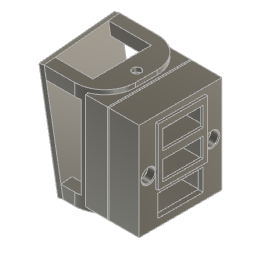
Lock Shoot v26 (Autodesk Fusion 360 design; units mm, degrees)
Autodesk Fusion 360 part; units mm, degrees
note: some values were not read from the file. Chosen so that the rebuilt part matches the saved one: which bodies a step acts on; which sketch regions a step uses; which face or edge a step refers to.
sketch "Sketch1" plane through (0, 0, 0) normal (1, 0, 0) x (0, 1, 0)
  line L0 (16, -20) -> (-16, -20)
  line L1 (-16, -20) -> (-16, 20)
  line L2 (-16, 20) -> (16, 20)
  line L3 (16, 20) -> (16, -20)
  line L4 (16, -20) -> (-16, 20) construction
  line L5 (-16, -20) -> (16, 20) construction
  line L6 (13, -0.5) -> (-13, -0.5)
  line L7 (-13, -0.5) -> (-13, 0.5)
  line L8 (-13, 0.5) -> (13, 0.5)
  line L9 (13, 0.5) -> (13, -0.5)
  line L10 (13, -0.5) -> (-13, 0.5) construction
  line L11 (-13, -0.5) -> (13, 0.5) construction
  circle A0 centre (13, 0) radius 1.6
  circle A1 centre (-13, 0) radius 1.6
  circle A2 centre (13, 0) radius 2.5
  circle A3 centre (-13, 0) radius 2.5
  line L12 (9.8559, -5.7872) -> (-9.8471, -5.7872)
  line L13 (-9.8471, -5.7872) -> (-9.8471, 17.1997)
  line L14 (-9.8471, 17.1997) -> (9.8559, 17.1997)
  line L15 (9.8559, 17.1997) -> (9.8559, -5.7872)
  line L16 (9.8559, -5.7872) -> (-9.8471, 17.1997) construction
  line L17 (-9.8471, -5.7872) -> (9.8559, 17.1997) construction
  line L18 (8.3025, -3.9749) -> (-8.3025, -3.9749)
  line L19 (-8.3025, -3.9749) -> (-8.3025, 3.9749)
  line L20 (-8.3025, 3.9749) -> (8.3025, 3.9749)
  line L21 (8.3025, 3.9749) -> (8.3025, -3.9749)
  line L22 (8.3025, -3.9749) -> (-8.3025, 3.9749) construction
  line L23 (-8.3025, -3.9749) -> (8.3025, 3.9749) construction
  line L24 (-8.3025, 7.0251) -> (-8.3025, 14.9749)
  line L25 (-8.3025, 14.9749) -> (8.3025, 14.9749)
  line L26 (8.3025, 14.9749) -> (8.3025, 7.0251)
  line L27 (8.3025, 7.0251) -> (-8.3025, 7.0251)
  line L28 (-9.3025, -8.0251) -> (9.3025, -8.0251)
  line L29 (-9.3025, -16.9749) -> (-9.3025, -8.0251)
  line L30 (9.3025, -16.9749) -> (-9.3025, -16.9749)
  line L31 (9.3025, -8.0251) -> (9.3025, -16.9749)
  line L32 (-8.3025, 14.9749) -> (-3.8025, 14.9749)
  line L33 (-3.8025, 14.9749) -> (-3.8025, 11)
  line L34 (-3.8025, 11) -> (-8.3025, 11)
  line L35 (-8.3025, 11) -> (-8.3025, 14.9749)
  line L36 (8.3025, 14.9749) -> (3.8025, 14.9749)
  line L37 (3.8025, 14.9749) -> (3.8025, 11)
  line L38 (3.8025, 11) -> (8.3025, 11)
  line L39 (8.3025, 11) -> (8.3025, 14.9749)
  circle A4 centre (-3.8025, 11) radius 2.5
  circle A5 centre (3.8025, 11) radius 2.5
  circle A6 centre (-3.8025, 0) radius 2.5
  circle A7 centre (3.8025, 0) radius 2.5
  line L40 (-9.3025, -8.0251) -> (-4.2025, -8.0251)
  line L41 (-4.2025, -8.0251) -> (-4.2025, -12.5)
  line L42 (-4.2025, -12.5) -> (-9.3025, -12.5)
  line L43 (-9.3025, -12.5) -> (-9.3025, -8.0251)
  line L44 (9.3025, -8.0251) -> (4.2025, -8.0251)
  line L45 (4.2025, -8.0251) -> (4.2025, -12.5)
  line L46 (4.2025, -12.5) -> (9.3025, -12.5)
  line L47 (9.3025, -12.5) -> (9.3025, -8.0251)
  circle A8 centre (-4.2025, -12.5) radius 2.5
  circle A9 centre (4.2025, -12.5) radius 2.55
  circle A10 centre (-13, 0) radius 2.85
  circle A11 centre (13, 0) radius 2.85
  point P0 (0.0044, 5.7062)
  dimension "d1" = 32
  dimension "d2" = 40
  dimension "d3" = 26
  dimension "d4" = 1
  dimension "d5" = 3.2
  dimension "d6" = 3.2
  dimension "d7" = 5
  dimension "d8" = 5
  dimension "d9" = 4.5
  dimension "d10" = 4.5
  dimension "d11" = 5
  dimension "d12" = 5
  dimension "d13" = 5
  dimension "d14" = 5
  dimension "d15" = 5.1
  dimension "d16" = 5.1
  dimension "d17" = 5
  dimension "d18" = 5.1
  dimension "d82" = 5.7
  dimension "d83" = 5.7
  constraint horizontal L0
  constraint perpendicular L0 L1
  constraint parallel L0 L2
  constraint parallel L1 L3
  constraint coincident L4 origin
  constraint coincident L5 origin
  constraint horizontal L6
  constraint perpendicular L6 L7
  constraint parallel L6 L8
  constraint parallel L7 L9
  constraint coincident L10 origin
  constraint coincident L11 origin
  constraint midpoint L9 A0.centre
  constraint midpoint L7 A1.centre
  constraint concentric A0 A2
  constraint concentric A1 A3
  constraint horizontal L12
  constraint perpendicular L12 L13
  constraint parallel L12 L14
  constraint parallel L13 L15
  constraint coincident L16 P0
  constraint coincident L17 P0
  constraint horizontal L18
  constraint perpendicular L18 L19
  constraint parallel L18 L20
  constraint parallel L19 L21
  constraint coincident L16 L18.start
  constraint coincident L22 origin
  constraint coincident L23 origin
  constraint horizontal L27
  constraint perpendicular L24 L27
  constraint parallel L25 L27
  constraint parallel L24 L26
  constraint horizontal L30
  constraint perpendicular L29 L30
  constraint parallel L28 L30
  constraint parallel L29 L31
  constraint horizontal L32
  constraint vertical L33
  constraint horizontal L34
  constraint vertical L35
  constraint horizontal L36
  constraint vertical L37
  constraint horizontal L38
  constraint vertical L39
  constraint coincident L33.end L34.start
  constraint coincident L37.end L38.start
  constraint horizontal L40
  constraint vertical L41
  constraint horizontal L42
  constraint vertical L43
  constraint horizontal L44
  constraint vertical L45
  constraint horizontal L46
  constraint vertical L47
  constraint coincident L41.end L42.start
  constraint coincident L45.end L46.start
  constraint concentric A1 A10
  constraint concentric A0 A11
  measures "d1" distance of L1.end L2.end
  measures "d2" distance of L0.end L1.end
  measures "d3" distance of L7.end L8.end
  measures "d4" distance of L6.end L7.end
  measures "d5" diameter of A0
  measures "d6" diameter of A1
  measures "d7" diameter of A2
  measures "d8" diameter of A3
  measures "d9" distance of L24.end L32.end
  measures "d10" distance of L25.end L36.end
  measures "d11" diameter of A4
  measures "d12" diameter of A5
  measures "d13" diameter of A6
  measures "d14" diameter of A7
  measures "d15" distance of L28.start L40.end
  measures "d16" distance of L28.end L44.end
  measures "d17" diameter of A8
  measures "d18" diameter of A9
  measures "d82" diameter of A10
  measures "d83" diameter of A11
extrude "Extrude1" add sketch "Sketch1" against normal blind 8 contours L0 L1 L2 L3 | L6 L8 A0 A2 | L6 L8 A0 A2 | L6 L8 A2 A11 | L6 L8 A2 A11 | L6 L8 L15 A11 | L6 L8 L13 A10 | L6 L8 A3 A10 | L6 L8 A3 A10 | L6 L8 A1 A3 | L6 L8 A1 A3 makes body 1
extrude "Extrude2" add sketch "Sketch1" along normal blind 1 separate body contours L6 L12 L13 L15 L18 L19 L21 | L6 L8 L15 L21 | L8 L13 L14 L15 L19 L20 L21 | L6 L8 L13 L19 makes body 2
sketch "Sketch2" plane through (-8, 0, 0) normal (-1, 0, 0) x (0, -1, 0)
  circle A0 centre (-13, 0) radius 1.6
  line L0 (-9.3025, -16.9749) -> (-9.3025, -8.0251)
  line L1 (-9.3025, -8.0251) -> (9.3025, -8.0251)
  line L2 (9.3025, -8.0251) -> (9.3025, -16.9749)
  line L3 (9.3025, -16.9749) -> (-9.3025, -16.9749)
  circle A1 centre (13, 0) radius 1.6
  line L4 (-9.8559, 17.1997) -> (9.8471, 17.1997)
  line L5 (9.8471, 17.1997) -> (9.8471, -5.7872)
  line L6 (9.8471, -5.7872) -> (-9.8559, -5.7872)
  line L7 (-9.8559, -5.7872) -> (-9.8559, 17.1997)
  line L8 (16, 20) -> (-16, 20)
  line L9 (-16, 20) -> (-16, -20)
  line L10 (-16, -20) -> (16, -20)
  line L11 (16, -20) -> (16, 20)
  line L12 (-10.5, -7) -> (10.5, -7)
  line L13 (10.5, -7) -> (10.5, -18)
  line L14 (10.5, -18) -> (-10.5, -18)
  line L15 (-10.5, -18) -> (-10.5, -7)
  line L16 (-10.5, -7) -> (10.5, -18) construction
  line L17 (10.5, -7) -> (-10.5, -18) construction
  line L18 (10, 6.5062) -> (-10, 6.5062)
  line L19 (-10, 6.5062) -> (-10, 4.9062)
  line L20 (-10, 4.9062) -> (10, 4.9062)
  line L21 (10, 4.9062) -> (10, 6.5062)
  line L22 (10, 6.5062) -> (-10, 4.9062) construction
  line L23 (-10, 6.5062) -> (10, 4.9062) construction
  line L24 (8.5, 15.45) -> (-8.5, 15.45)
  line L25 (-8.5, 15.45) -> (-8.5, -15.45)
  line L26 (-8.5, -15.45) -> (8.5, -15.45)
  line L27 (8.5, -15.45) -> (8.5, 15.45)
  line L28 (8.5, 15.45) -> (-8.5, -15.45) construction
  line L29 (-8.5, 15.45) -> (8.5, -15.45) construction
  point P0 (0, -12.5)
  point P1 (0, 5.7062)
  dimension "d23" = 21
  dimension "d24" = 11
  dimension "d25" = 20
  dimension "d26" = 1.6
  dimension "d31" = 17
  dimension "d32" = 30.9
  constraint horizontal L12
  constraint perpendicular L12 L13
  constraint parallel L12 L14
  constraint parallel L13 L15
  constraint coincident L16 P0
  constraint coincident L17 P0
  constraint horizontal L18
  constraint perpendicular L18 L19
  constraint parallel L18 L20
  constraint parallel L19 L21
  constraint coincident L22 P1
  constraint coincident L23 P1
  constraint horizontal L24
  constraint perpendicular L24 L25
  constraint parallel L24 L26
  constraint parallel L25 L27
  constraint coincident L28 origin
  constraint coincident L29 origin
  measures "d23" distance of L13.end L14.end
  measures "d24" distance of L12.end L13.end
  measures "d25" distance of L19.end L20.end
  measures "d26" distance of L18.end L19.end
  measures "d31" distance of L25.end L26.end
  measures "d32" distance of L24.end L25.end
extrude "Extrude3" add sketch "Sketch2" against normal blind 8 contours L18 L20 L25 L27 | L7 L18 L20 L25 | L5 L18 L20 L27 bodies 1 2
extrude "Extrude4" cut sketch "Sketch2" against normal blind 6 contours L0 L1 L2 L3 L12 L13 L14 L15 L25 L27 | L1 L12 L25 L27 bodies 1
sketch "Sketch3" plane through (-8, 0, 0) normal (-1, 0, 0) x (0, 1, 0)
extrude "Extrude5" cut sketch "Sketch2" against normal blind 1.6 contours L6 L12 L25 L27 | L18 L20 L25 L27 bodies 1
sketch "Sketch4" plane through (-6.4, 0, 0) normal (-1, 0, 0) x (0, -1, 0)
  line L0 (-8.5, 4.9062) -> (8.5, 4.9062)
  line L1 (8.5, 4.9062) -> (8.5, 6.5062)
  line L2 (8.5, 6.5062) -> (-8.5, 6.5062)
  line L3 (-8.5, 6.5062) -> (-8.5, 4.9062)
  line L4 (4.5068, 3.4673) -> (-4.4932, 3.4673)
  line L5 (-4.4932, 3.4673) -> (-4.4932, 7.9579)
  line L6 (-4.4932, 7.9579) -> (4.5068, 7.9579)
  line L7 (4.5068, 7.9579) -> (4.5068, 3.4673)
  line L8 (4.5068, 3.4673) -> (-4.4932, 7.9579) construction
  line L9 (-4.4932, 3.4673) -> (4.5068, 7.9579) construction
  point P0 (0.0068, 5.7126)
  dimension "d35" = 9
  constraint horizontal L4
  constraint perpendicular L4 L5
  constraint parallel L4 L6
  constraint parallel L5 L7
  constraint coincident L8 P0
  constraint coincident L9 P0
  measures "d35" distance of L5.end L6.end
extrude "Extrude6" cut sketch "Sketch4" against normal blind 2 contours L0 L2 L5 L7 bodies 1
extrude "Extrude8" add 1 faces at (-8, -13.2157, 9.2973) along direction (-1, 0, 0) blind 3 on bodies 1 bodies 1
extrude "Extrude9" add 3 faces at (-6.4, -5.8379, 5.9729) (-6.4, 7.1644, 5.9729) (-6.4, 2.8333, -6.5957) along direction (-1, 0, 0) blind 3 on bodies 1 bodies 1
extrude "Extrude10" add 1 faces at (-4.4, 1.4932, 5.4395) along direction (-1, 0, 0) blind 3 on bodies 1 bodies 1
sketch "Sketch5" plane through (-9.4, 0, 0) normal (-1, 0, 0) x (0, -1, 0)
  line L0 (-8.5, -7) -> (8.5, -7)
  line L1 (8.5, -7) -> (8.5, -5.7872)
  line L2 (8.5, -5.7872) -> (-8.5, -5.7872)
  line L3 (-8.5, -5.7872) -> (-8.5, -7)
  circle A0 centre (0, -6.3723) radius 1.4
  dimension "d60" = 2.8
  measures "d60" diameter of A0
extrude "Extrude11" cut sketch "Sketch5" against normal blind 2.8 contours L0 L2 A0 bodies 1
extrude "Extrude12" add 1 faces at (0.6667, -9.8471, 5.4395) along direction (0, -1, 0) blind 0.3 on bodies 1 bodies 1
extrude "Extrude13" add 1 faces at (0.6667, -3.3794, 17.1997) along direction (0, 0, 1) blind 0.3 on bodies 1 bodies 1
extrude "Extrude14" add 2 faces at (0.6667, 9.8559, 5.4395) (0.3333, 9.8559, 17.2997) along direction (0, 1, 0) blind 0.3 on bodies 1 bodies 1
extrude "Extrude15" add 1 faces at (0.6667, 3.2883, -5.7872) along direction (0, 0, -1) blind 0.3 on bodies 1 bodies 1
sketch "Sketch6" plane through (-11, 0, 0) normal (-1, 0, 0) x (0, -1, 0)
  line L0 (16, 20) -> (-16, 20)
  line L1 (-16, 20) -> (-16, -20)
  line L2 (-16, -20) -> (16, -20)
  line L3 (16, -20) -> (16, 20)
  circle A0 centre (13, 0) radius 1.6
  circle A1 centre (-13, 0) radius 1.6
  line L4 (8.5, 6.5062) -> (8.5, 4.9062)
  line L5 (8.5, 4.9062) -> (9.8471, 4.9062)
  line L6 (9.8471, 4.9062) -> (9.8471, -5.7872)
  line L7 (9.8471, -5.7872) -> (8.5, -5.7872)
  line L8 (8.5, -5.7872) -> (8.5, -7)
  line L9 (8.5, -7) -> (10.5, -7)
  line L10 (10.5, -7) -> (10.5, -18)
  line L11 (10.5, -18) -> (-10.5, -18)
  line L12 (-10.5, -18) -> (-10.5, -7)
  line L13 (-10.5, -7) -> (-8.5, -7)
  line L14 (-8.5, -7) -> (-8.5, -5.7872)
  line L15 (-8.5, -5.7872) -> (-9.8559, -5.7872)
  line L16 (-9.8559, -5.7872) -> (-9.8559, 4.9062)
  line L17 (-9.8559, 4.9062) -> (-8.5, 4.9062)
  line L18 (-8.5, 4.9062) -> (-8.5, 6.5062)
  line L19 (-8.5, 6.5062) -> (-9.8559, 6.5062)
  line L20 (-9.8559, 6.5062) -> (-9.8559, 17.1997)
  line L21 (-9.8559, 17.1997) -> (9.8471, 17.1997)
  line L22 (9.8471, 17.1997) -> (9.8471, 6.5062)
  line L23 (9.8471, 6.5062) -> (8.5, 6.5062)
  circle A2 centre (-0.001, -6.3625) radius 1.6
  line L24 (6.2705, 2.0911) -> (-6.2754, 2.0911)
  line L25 (-6.2754, 2.0911) -> (-6.2754, 9.3782)
  line L26 (-6.2754, 9.3782) -> (6.2705, 9.3782)
  line L27 (6.2705, 9.3782) -> (6.2705, 2.0911)
  line L28 (6.2705, 2.0911) -> (-6.2754, 9.3782) construction
  line L29 (-6.2754, 2.0911) -> (6.2705, 9.3782) construction
  point P0 (-0.0025, 5.7347)
  dimension "d57" = 3.2
  constraint horizontal L24
  constraint perpendicular L24 L25
  constraint parallel L24 L26
  constraint parallel L25 L27
  constraint coincident L28 P0
  constraint coincident L29 P0
  measures "d57" diameter of A2
extrude "Extrude16" add 1 faces at (-6.6, 0.3936, -6.2542) along direction (-1, 0, 0) blind 2.8 on bodies 1 bodies 1
extrude "Extrude17" add sketch "Sketch5" along normal blind 1.6 contours L0 L2 A0 | L0 A0 | L2 A0 bodies 1
extrude "Extrude18" add 1 faces at (-11, -13.2157, 9.2973) along direction (-1, 0, 0) blind 10 separate body on bodies 1 makes body 3
sketch "Sketch7" plane through (-21, 0, 0) normal (-1, 0, 0) x (0, -1, 0)
  line L0 (16, 20) -> (-16, 20)
  line L1 (-16, 20) -> (-16, -20)
  line L2 (-16, -20) -> (16, -20)
  line L3 (16, -20) -> (16, 20)
  circle A0 centre (13, 0) radius 1.6
  circle A1 centre (-13, 0) radius 1.6
  line L4 (8.5, 6.5062) -> (8.5, 4.9062)
  line L5 (8.5, 4.9062) -> (9.8471, 4.9062)
  line L6 (9.8471, 4.9062) -> (9.8471, -5.7872)
  line L7 (9.8471, -5.7872) -> (8.5, -5.7872)
  line L8 (8.5, -5.7872) -> (8.5, -7)
  line L9 (8.5, -7) -> (10.5, -7)
  line L10 (10.5, -7) -> (10.5, -18)
  line L11 (10.5, -18) -> (-10.5, -18)
  line L12 (-10.5, -18) -> (-10.5, -7)
  line L13 (-10.5, -7) -> (-8.5, -7)
  line L14 (-8.5, -7) -> (-8.5, -5.7872)
  line L15 (-8.5, -5.7872) -> (-9.8559, -5.7872)
  line L16 (-9.8559, -5.7872) -> (-9.8559, 4.9062)
  line L17 (-9.8559, 4.9062) -> (-8.5, 4.9062)
  line L18 (-8.5, 4.9062) -> (-8.5, 6.5062)
  line L19 (-8.5, 6.5062) -> (-9.8559, 6.5062)
  line L20 (-9.8559, 6.5062) -> (-9.8559, 17.1997)
  line L21 (-9.8559, 17.1997) -> (9.8471, 17.1997)
  line L22 (9.8471, 17.1997) -> (9.8471, 6.5062)
  line L23 (9.8471, 6.5062) -> (8.5, 6.5062)
  line L24 (16, -20) -> (-16, -20)
  line L25 (-16, -20) -> (-16, 20)
  line L26 (-16, 20) -> (16, 20)
  line L27 (16, 20) -> (16, -20)
  line L28 (16, -20) -> (-16, 20) construction
  line L29 (-16, -20) -> (16, 20) construction
  line L30 (-10.2309, -1.6038) -> (-10.2265, 1.5962)
  line L31 (-10.2265, 1.5962) -> (-12.9956, 3.2)
  line L32 (-12.9956, 3.2) -> (-15.7691, 1.6038)
  line L33 (-15.7691, 1.6038) -> (-15.7735, -1.5962)
  line L34 (-15.7735, -1.5962) -> (-13.0044, -3.2)
  line L35 (-13.0044, -3.2) -> (-10.2309, -1.6038)
  line L36 (13.0326, -3.1998) -> (15.7875, -1.5717)
  line L37 (15.7875, -1.5717) -> (15.7548, 1.6282)
  line L38 (15.7548, 1.6282) -> (12.9674, 3.1998)
  line L39 (12.9674, 3.1998) -> (10.2125, 1.5717)
  line L40 (10.2125, 1.5717) -> (10.2452, -1.6282)
  line L41 (10.2452, -1.6282) -> (13.0326, -3.1998)
  point P0 (-13, 0)
  point P1 (13, 0)
  dimension "d76" = 3.2
  dimension "d77" = 3.2
  constraint horizontal L24
  constraint perpendicular L24 L25
  constraint parallel L24 L26
  constraint parallel L25 L27
  constraint coincident L2.end L3.start
  constraint coincident L28 origin
  constraint coincident L29 origin
  constraint coincident P0 A1.centre
  constraint coincident P1 A0.centre
  measures "d76" distance of L30.start P0
  measures "d77" distance of L36.start P1
extrude "Extrude19" add sketch "Sketch7" along normal blind 1 contours L0 L1 L2 L3 L24 L25 L26 L27 | L4 L5 L6 L7 L8 L9 L10 L11 L12 L13 L14 L15 L16 L17 L18 L19 L20 L21 L22 L23 | L30 L31 L32 L33 L34 L35 | L36 L37 L38 L39 L40 L41 bodies 3
sketch "Sketch8" plane through (-11, 0, 0) normal (1, 0, 0) x (0, 1, 0)
  line L0 (16, 20) -> (-16, 20)
  line L1 (-16, 20) -> (-16, -20)
  line L2 (-16, -20) -> (16, -20)
  line L3 (16, -20) -> (16, 20)
  circle A0 centre (-13, 0) radius 1.6
  circle A1 centre (13, 0) radius 1.6
  line L4 (-8.5, 4.9062) -> (-8.5, 6.5062)
  line L5 (-8.5, 6.5062) -> (-9.8471, 6.5062)
  line L6 (-9.8471, 6.5062) -> (-9.8471, 17.1997)
  line L7 (-9.8471, 17.1997) -> (9.8559, 17.1997)
  line L8 (9.8559, 17.1997) -> (9.8559, 6.5062)
  line L9 (9.8559, 6.5062) -> (8.5, 6.5062)
  line L10 (8.5, 6.5062) -> (8.5, 4.9062)
  line L11 (8.5, 4.9062) -> (9.8559, 4.9062)
  line L12 (9.8559, 4.9062) -> (9.8559, -5.7872)
  line L13 (9.8559, -5.7872) -> (8.5, -5.7872)
  line L14 (8.5, -5.7872) -> (8.5, -7)
  line L15 (8.5, -7) -> (10.5, -7)
  line L16 (10.5, -7) -> (10.5, -18)
  line L17 (10.5, -18) -> (-10.5, -18)
  line L18 (-10.5, -18) -> (-10.5, -7)
  line L19 (-10.5, -7) -> (-8.5, -7)
  line L20 (-8.5, -7) -> (-8.5, -5.7872)
  line L21 (-8.5, -5.7872) -> (-9.8471, -5.7872)
  line L22 (-9.8471, -5.7872) -> (-9.8471, 4.9062)
  line L23 (-9.8471, 4.9062) -> (-8.5, 4.9062)
  line L24 (16, -20) -> (-16, -20)
  line L25 (-16, -20) -> (-16, 20)
  line L26 (-16, 20) -> (16, 20)
  line L27 (16, 20) -> (16, -20)
  line L28 (16, -20) -> (-16, 20) construction
  line L29 (-16, -20) -> (16, 20) construction
  constraint horizontal L24
  constraint perpendicular L24 L25
  constraint parallel L24 L26
  constraint parallel L25 L27
  constraint coincident L2.end L3.start
  constraint coincident L28 origin
  constraint coincident L29 origin
extrude "Extrude20" add sketch "Sketch8" against normal blind 2 contours L4 L5 L6 L7 L8 L9 L10 L11 L12 L13 L14 L15 L16 L17 L18 L19 L20 L21 L22 L23 bodies 3
sketch "Sketch9" plane through (-7.4, 0, 0) normal (-1, 0, 0) x (0, -1, 0)
  line L0 (-4.4932, 4.9062) -> (4.5068, 4.9062)
  line L1 (4.5068, 4.9062) -> (4.5068, 6.5062)
  line L2 (4.5068, 6.5062) -> (-4.4932, 6.5062)
  line L3 (-4.4932, 6.5062) -> (-4.4932, 4.9062)
  line L4 (-5.9932, 9.7062) -> (6.0068, 9.7062)
  line L5 (6.0068, 9.7062) -> (6.0068, -2.2938)
  line L6 (6.0068, -2.2938) -> (-5.9932, -2.2938)
  line L7 (-5.9932, -2.2938) -> (-5.9932, 9.7062)
  line L8 (-5.9932, 9.7062) -> (6.0068, -2.2938) construction
  line L9 (6.0068, 9.7062) -> (-5.9932, -2.2938) construction
  circle A0 centre (0.0068, 3.7062) radius 4
  point P0 (0.0068, 3.7062)
  dimension "d69" = 12
  dimension "d70" = 12
  dimension "d73" = 8
  constraint horizontal L4
  constraint perpendicular L4 L5
  constraint parallel L4 L6
  constraint parallel L5 L7
  constraint coincident L8 P0
  constraint coincident L9 P0
  constraint coincident P0 A0.centre
  measures "d69" distance of L5.end L6.end
  measures "d70" distance of L4.end L5.end
  measures "d73" diameter of A0
extrude "Extrude21" cut sketch "Sketch9" along normal blind 13 contours L0 L2 L3 A0 | L0 L2 A0 | L0 A0 | L0 L1 L2 A0 | L2 A0 | L4 L5 L6 L7 bodies 1 3
extrude "Extrude22" cut sketch "Sketch9" along normal blind 31 contours L0 L2 A0 | L0 A0 | L2 A0 bodies 3
extrude "Extrude23" cut sketch "Sketch7" along normal blind 2 and the other way blind 8 contours A0 | A1 | L30 L31 L32 L33 L34 L35 | L36 L37 L38 L39 L40 L41 bodies 3
extrude "Extrude24" cut sketch "Sketch1" against normal blind 3.3 contours L6 L8 A0 A2 | L6 L8 A0 A2 | L6 L8 A2 A11 | L6 L8 A2 A11 | L6 L8 A3 A10 | L6 L8 A3 A10 | L6 L8 A1 A3 | L6 L8 A1 A3 bodies 1
move_face "OffsetFaces1" offset 0.5 1 faces at (-7.3333, -16, 6.6667) on bodies 1
move_face "OffsetFaces2" offset 0.5 1 faces at (-14.6667, -16, -6.6667) on bodies 3
move_face "OffsetFaces3" offset 0.5 1 faces at (-3.6667, 16, 6.6667) on bodies 1
move_face "OffsetFaces4" offset 0.5 1 faces at (-14.6667, 16, 6.6667) on bodies 3
sketch "Sketch10" plane through (-11, 0, 0) normal (-1, 0, 0) x (0, -1, 0)
  line L0 (16.5, 20) -> (-16.5, 20)
  line L1 (-16.5, 20) -> (-16.5, -20)
  line L2 (-16.5, -20) -> (16.5, -20)
  line L3 (16.5, -20) -> (16.5, 20)
  circle A0 centre (-13, 0) radius 1.6
  circle A1 centre (13, 0) radius 1.6
  line L4 (8.5, 6.5062) -> (8.5, 4.9062)
  line L5 (8.5, 4.9062) -> (9.8471, 4.9062)
  line L6 (9.8471, 4.9062) -> (9.8471, -5.7872)
  line L7 (9.8471, -5.7872) -> (8.5, -5.7872)
  line L8 (8.5, -5.7872) -> (8.5, -7)
  line L9 (8.5, -7) -> (10.5, -7)
  line L10 (10.5, -7) -> (10.5, -18)
  line L11 (10.5, -18) -> (-10.5, -18)
  line L12 (-10.5, -18) -> (-10.5, -7)
  line L13 (-10.5, -7) -> (-8.5, -7)
  line L14 (-8.5, -7) -> (-8.5, -5.7872)
  line L15 (-8.5, -5.7872) -> (-9.8559, -5.7872)
  line L16 (-9.8559, -5.7872) -> (-9.8559, 4.9062)
  line L17 (-9.8559, 4.9062) -> (-8.5, 4.9062)
  line L18 (-8.5, 4.9062) -> (-8.5, 6.5062)
  line L19 (-8.5, 6.5062) -> (-9.8559, 6.5062)
  line L20 (-9.8559, 6.5062) -> (-9.8559, 17.1997)
  line L21 (-9.8559, 17.1997) -> (9.8471, 17.1997)
  line L22 (9.8471, 17.1997) -> (9.8471, 6.5062)
  line L23 (9.8471, 6.5062) -> (8.5, 6.5062)
  line L24 (-16.5, -20) -> (16.5, -20)
  line L25 (16.5, -20) -> (16.5, 20)
  line L26 (16.5, 20) -> (-16.5, 20)
  line L27 (-16.5, 20) -> (-16.5, -20)
  line L28 (-16.5, -20) -> (16.5, 20) construction
  line L29 (16.5, -20) -> (-16.5, 20) construction
  line L30 (-15.5, -19) -> (15.5, -19)
  line L31 (15.5, -19) -> (15.5, 19)
  line L32 (15.5, 19) -> (-15.5, 19)
  line L33 (-15.5, 19) -> (-15.5, -19)
  line L34 (-15.5, -19) -> (15.5, 19) construction
  line L35 (15.5, -19) -> (-15.5, 19) construction
  line L36 (4.5, 1.5956) -> (-4.5, 1.5956)
  line L37 (-4.5, 1.5956) -> (-4.5, 10.5956)
  line L38 (-4.5, 10.5956) -> (4.5, 10.5956)
  line L39 (4.5, 10.5956) -> (4.5, 1.5956)
  line L40 (4.5, 1.5956) -> (-4.5, 10.5956) construction
  line L41 (-4.5, 1.5956) -> (4.5, 10.5956) construction
  point P0 (0, 6.0956)
  dimension "d90" = 31
  dimension "d91" = 38
  dimension "d104" = 9
  dimension "d105" = 9
  constraint horizontal L24
  constraint perpendicular L24 L25
  constraint parallel L24 L26
  constraint parallel L25 L27
  constraint coincident L1.end L2.start
  constraint coincident L28 origin
  constraint coincident L29 origin
  constraint horizontal L30
  constraint perpendicular L30 L31
  constraint parallel L30 L32
  constraint parallel L31 L33
  constraint coincident L34 origin
  constraint coincident L35 origin
  constraint horizontal L36
  constraint perpendicular L36 L37
  constraint parallel L36 L38
  constraint parallel L37 L39
  constraint coincident L40 P0
  constraint coincident L41 P0
  measures "d90" distance of L31.end L32.end
  measures "d91" distance of L30.end L31.end
  measures "d104" distance of L37.end L38.end
  measures "d105" distance of L36.end L37.end
extrude "Extrude25" add sketch "Sketch10" along normal blind 2 contours L0 L1 L2 L3 L24 L25 L26 L27 bodies 1
extrude "Extrude26" cut sketch "Sketch10" along normal blind 1.9 contours L0 L1 L2 L3 L24 L25 L26 L27 bodies 3
fillet "Fillet1" radius 0.5 8 edges at (-11.95, -15.5, 19) (-11.95, -15.5, -19) (-11.95, 15.5, 19) (-11.95, 15.5, -19) (-11, 15.5, 0) (-11, 0, 19) (-11, -15.5, 0) (-11, 0, -19) on bodies 3
fillet "Fillet2" radius 0.3 2 edges at (0, -15.6571, 1.0306) (0, 15.85, 0) on bodies 1
move_face "OffsetFaces5" offset 0.5 1 faces at (-4.3333, -16.5, -6.6667) on bodies 1
move_face "OffsetFaces6" offset 0.5 1 faces at (-15.9333, -16.5, -6.6667) on bodies 3
move_face "OffsetFaces7" offset 0.5 1 faces at (-8.6667, 16.5, -6.6667) on bodies 1
move_face "OffsetFaces8" offset 0.5 1 faces at (-15.9333, 16.5, 6.6667) on bodies 3
extrude "Extrude27" cut sketch "Sketch10" along normal blind 20 contours L36 L37 L38 L39 bodies 3
sketch "Sketch11" plane through (-11, 0, 0) normal (1, 0, 0) x (0, 1, 0)
  circle A0 centre (-13, 0) radius 1.6
  circle A1 centre (13, 0) radius 1.6
  line L0 (5.9932, 9.7062) -> (5.9932, -2.2938)
  line L1 (5.9932, -2.2938) -> (-6.0068, -2.2938)
  line L2 (-6.0068, -2.2938) -> (-6.0068, 9.7062)
  line L3 (4.5, 9.7062) -> (5.9932, 9.7062)
  line L4 (-15, -18.5) -> (15, -18.5)
  line L5 (15, -18.5) -> (15, 18.5)
  line L6 (15, 18.5) -> (-15, 18.5)
  line L7 (-15, 18.5) -> (-15, -18.5)
  line L8 (-4.5, 9.7062) -> (-4.5, 10.5956)
  line L9 (-4.5, 10.5956) -> (4.5, 10.5956)
  line L10 (4.5, 10.5956) -> (4.5, 9.7062)
  line L11 (-6.0068, 9.7062) -> (-4.5, 9.7062)
sketch "Sketch12" plane through (-11, 0, 0) normal (1, 0, 0) x (0, 1, 0)
  line L0 (0, 0) -> (0, -12)
  line L1 (6.5, -13.5) -> (-6.5, -13.5)
  line L2 (-6.5, -13.5) -> (-6.5, -10.5)
  line L3 (-6.5, -10.5) -> (6.5, -10.5)
  line L4 (6.5, -10.5) -> (6.5, -13.5)
  line L5 (6.5, -13.5) -> (-6.5, -10.5) construction
  line L6 (-6.5, -13.5) -> (6.5, -10.5) construction
  point P0 (0, -12)
  dimension "d108" = 12
  dimension "d109" = 13
  dimension "d110" = 3
  constraint coincident L0.start origin
  constraint vertical L0
  constraint horizontal L1
  constraint perpendicular L1 L2
  constraint parallel L1 L3
  constraint parallel L2 L4
  constraint coincident L5 P0
  constraint coincident L6 P0
  constraint coincident P0 L0.end
  measures "d108" distance of L0.start P0
  measures "d109" distance of L2.end L3.end
  measures "d110" distance of L1.end L2.end
extrude "Extrude28" cut sketch "Sketch12" against normal blind 3 bodies 3
sketch "Sketch13" plane through (-11, 0, 0) normal (1, 0, 0) x (0, 1, 0)
  circle A0 centre (0.0016, -6.3729) radius 1.3995
extrude "Extrude29" add sketch "Sketch13" along normal blind 2.2 bodies 3
extrude "Extrude30" add 1 faces at (-12.9, 16.5, -6.1667) along direction (1, 0, 0) blind 0.5 on bodies 3 bodies 3
delete_face "DeleteFace1" 1 faces at (-21.6667, 2.7872, 0.8438) on bodies 3
extrude "Extrude31" cut 2 faces at (-12.3333, -5.5046, 9.7062) (-12.3333, 4.9977, 9.7062) along direction (0, 0, 1) blind 3.5 on bodies 3 bodies 3
extrude "Extrude32" cut 1 faces at (-12.3333, 1.5, 10.5956) along direction (0, 0, 1) blind 2.611 on bodies 3 bodies 3
extrude "Extrude33" cut 1 faces at (-11, -0.0739, -6.1161) along direction (1, 0, 0) blind 1.6 on bodies 1 bodies 1
sketch "Sketch14" plane through (0, 0, 20) normal (0, 0, 1) x (-1, 0, 0)
  line L0 (12.4, -17) -> (22, -17)
  line L1 (22, -17) -> (22, 17)
  line L2 (22, 17) -> (12.4, 17)
  line L3 (12.4, 17) -> (12.4, -17)
  line L4 (12.4, -17) -> (22, 17)
  line L5 (22, -17) -> (12.4, 17)
  line L6 (17.2, 0) -> (22, 0)
  line L7 (22, 0) -> (18, 0)
  circle A0 centre (18, 0) radius 2
  circle A1 centre (18, 0) radius 3.5
  dimension "d123" = 4
  dimension "d124" = 4
  dimension "d125" = 7
  constraint coincident L0.start L3.end
  constraint coincident L1.end L2.start
  constraint coincident L0.end L1.start
  constraint coincident L2.end L3.start
  constraint midpoint L5 L6.start
  constraint midpoint L1 L6.end
  constraint parallel L6 L7
  constraint coincident L7.end A0.centre
  constraint concentric A0 A1
  measures "d123" distance of L6.end L7.end
  measures "d124" diameter of A0
  measures "d125" diameter of A1
extrude "Extrude34" add sketch "Sketch14" against normal blind 7 contours L4 L5 A0 A1 | L4 L5 A0 A1 | L5 L6 L7 A0 A1 | L4 L5 A0 A1 | L4 L6 L7 A0 A1 bodies 3
extrude "Extrude35" cut sketch "Sketch14" against normal blind 7 contours L4 L5 A0 | L4 L5 A0 | L5 L6 L7 A0 | L4 L5 A0 | L4 L6 L7 A0 bodies 3
sketch "Sketch15" plane through (0, 0, -20) normal (0, 0, -1) x (1, 0, 0)
  line L0 (-12.4, 17) -> (-22, 17)
  line L1 (-22, 17) -> (-22, -17)
  line L2 (-22, -17) -> (-12.4, -17)
  line L3 (-12.4, -17) -> (-12.4, 17)
  line L4 (-22, 0) -> (-21.3553, 0)
  line L5 (-22, 0) -> (-18, 0)
  circle A0 centre (-18, 0) radius 2
  circle A1 centre (-18, 0) radius 3.5
  dimension "d130" = 4
  dimension "d131" = 4
  dimension "d132" = 7
  constraint midpoint L1 L4.start
  constraint perpendicular L1 L4
  constraint perpendicular L1 L5
  constraint coincident L5.end A0.centre
  constraint concentric A0 A1
  measures "d130" distance of L4.start L5.end
  measures "d131" diameter of A0
  measures "d132" diameter of A1
extrude "Extrude36" add sketch "Sketch15" against normal blind 7 contours A1 bodies 3
extrude "Extrude37" cut sketch "Sketch15" against normal blind 7 contours A0 bodies 3
extrude "Extrude38" cut 1 faces at (-18.3333, -8.5, 5.9729) along direction (0, -1, 0) blind 1.347 on bodies 3 bodies 3
extrude "Extrude39" cut 1 faces at (-18.3333, 8.5, 5.4395) along direction (0, 1, 0) blind 1.356 on bodies 3 bodies 3
extrude "Extrude40" cut 1 faces at (-18.3333, -8.5, -6.1915) along direction (0, -1, 0) blind 1.347 on bodies 3 bodies 3
extrude "Extrude41" cut 1 faces at (-18.3333, 8.5, -6.5957) along direction (0, 1, 0) blind 1.356 on bodies 3 bodies 3
copy_body "Body->Comp1" bodies 3 removing the originals makes body 4 in component "Rear"
copy_body "Body->Comp2" bodies 1 removing the originals makes body 5 in component "Front"
sketch "Sketch16" plane through (-22, 0, 0) normal (-1, 0, 0) x (0, -1, 0)
  line L0 (17, 20) -> (-17, 20)
  line L1 (-17, 20) -> (-17, -20)
  line L2 (-17, -20) -> (17, -20)
  line L3 (17, -20) -> (17, 20)
  line L4 (10.2452, -1.6282) -> (10.2125, 1.5717)
  line L5 (10.2125, 1.5717) -> (12.9674, 3.1998)
  line L6 (12.9674, 3.1998) -> (15.7548, 1.6282)
  line L7 (15.7548, 1.6282) -> (15.7875, -1.5717)
  line L8 (15.7875, -1.5717) -> (13.0326, -3.1998)
  line L9 (13.0326, -3.1998) -> (10.2452, -1.6282)
  line L10 (-13.0044, -3.2) -> (-15.7735, -1.5962)
  line L11 (-15.7735, -1.5962) -> (-15.7691, 1.6038)
  line L12 (-15.7691, 1.6038) -> (-12.9956, 3.2)
  line L13 (-12.9956, 3.2) -> (-10.2265, 1.5962)
  line L14 (-10.2265, 1.5962) -> (-10.2309, -1.6038)
  line L15 (-10.2309, -1.6038) -> (-13.0044, -3.2)
  line L16 (4.5, 1.5956) -> (-4.5, 1.5956)
  line L17 (-4.5, 1.5956) -> (-4.5, 10.5956)
  line L18 (-4.5, 10.5956) -> (4.5, 10.5956)
  line L19 (4.5, 10.5956) -> (4.5, 1.5956)
  line L20 (17, -22) -> (-17, -22)
  line L21 (-17, -22) -> (-17, 22)
  line L22 (-17, 22) -> (17, 22)
  line L23 (17, 22) -> (17, -22)
  line L24 (17, -22) -> (-17, 22) construction
  line L25 (-17, -22) -> (17, 22) construction
  line L26 (-17, -20) -> (17, -20)
  line L27 (17, -20) -> (17, -22)
  line L28 (17, -22) -> (-17, -22)
  line L29 (-17, -22) -> (-17, -20)
  line L30 (-17, 22) -> (17, 22)
  line L31 (17, 22) -> (17, 20)
  line L32 (17, 20) -> (-17, 20)
  line L33 (-17, 20) -> (-17, 22)
  line L34 (-4.5, 6.0956) -> (4.5, 6.0956)
  line L35 (7.664, -2.9908) -> (-7.664, -2.9908)
  line L36 (-7.664, -2.9908) -> (-7.664, 15.1819)
  line L37 (-7.664, 15.1819) -> (7.664, 15.1819)
  line L38 (7.664, 15.1819) -> (7.664, -2.9908)
  line L39 (7.664, -2.9908) -> (-7.664, 15.1819) construction
  line L40 (-7.664, -2.9908) -> (7.664, 15.1819) construction
  line L41 (-17, 22) -> (-12, 22)
  line L42 (-12, 22) -> (-12, 17)
  line L43 (-12, 17) -> (-17, 17)
  line L44 (-17, 17) -> (-17, 22)
  line L45 (17, 22) -> (12, 22)
  line L46 (12, 22) -> (12, 17)
  line L47 (12, 17) -> (17, 17)
  line L48 (17, 17) -> (17, 22)
  line L49 (17, -22) -> (12, -22)
  line L50 (12, -22) -> (12, -17)
  line L51 (12, -17) -> (17, -17)
  line L52 (17, -17) -> (17, -22)
  line L53 (-17, -22) -> (-12, -22)
  line L54 (-12, -22) -> (-12, -17)
  line L55 (-12, -17) -> (-17, -17)
  line L56 (-17, -17) -> (-17, -22)
  point P0 (0, 6.0956)
  dimension "d145" = 44
  dimension "d152" = 5
  dimension "d153" = 5
  dimension "d154" = 5
  dimension "d155" = 5
  dimension "d156" = 5
  dimension "d157" = 5
  dimension "d158" = 5
  dimension "d159" = 5
  constraint horizontal L20
  constraint perpendicular L20 L21
  constraint parallel L20 L22
  constraint parallel L21 L23
  constraint coincident L24 origin
  constraint coincident L25 origin
  constraint horizontal L26
  constraint vertical L27
  constraint horizontal L28
  constraint vertical L29
  constraint coincident L1.end L2.start
  constraint horizontal L30
  constraint vertical L31
  constraint horizontal L32
  constraint vertical L33
  constraint coincident L0.start L3.end
  constraint midpoint L17 L34.start
  constraint midpoint L19 L34.end
  constraint horizontal L35
  constraint perpendicular L35 L36
  constraint parallel L35 L37
  constraint parallel L36 L38
  constraint coincident L39 P0
  constraint coincident L40 P0
  constraint midpoint L34 P0
  constraint horizontal L41
  constraint vertical L42
  constraint horizontal L43
  constraint vertical L44
  constraint horizontal L45
  constraint vertical L46
  constraint horizontal L47
  constraint vertical L48
  constraint horizontal L49
  constraint vertical L50
  constraint horizontal L51
  constraint vertical L52
  constraint horizontal L53
  constraint vertical L54
  constraint horizontal L55
  constraint vertical L56
  measures "d145" distance of L20.end L21.end
  measures "d152" distance of L21.end L41.end
  measures "d153" distance of L21.end L43.end
  measures "d154" distance of L22.end L45.end
  measures "d155" distance of L22.end L47.end
  measures "d156" distance of L20.start L49.end
  measures "d157" distance of L20.start L51.end
  measures "d158" distance of L20.end L53.end
  measures "d159" distance of L20.end L55.end
extrude "Extrude1'" add sketch "Sketch16" against normal blind 8 separate body contours L0 L22 L23 L30 L31 L32 L45 L46 L48 | L0 L22 L30 L32 L42 L46 | L0 L21 L22 L30 L32 L33 L41 L42 L44 makes body 6 in component "Mount"
extrude "Extrude2'" add sketch "Sketch16" along normal blind 2 contours L0 L3 L23 L32 L46 L47 L48 | L0 L22 L23 L30 L31 L32 L45 L46 L48 | L0 L1 L2 L3 L21 L23 L26 L32 L42 L43 L46 L47 L50 L51 L54 L55 | L0 L22 L30 L32 L42 L46 | L0 L1 L21 L32 L42 L43 L44 | L0 L21 L22 L30 L32 L33 L41 L42 L44 | L2 L3 L23 L26 L50 L51 L52 | L2 L20 L23 L26 L27 L28 L49 L50 L52 | L2 L20 L26 L28 L50 L54 | L1 L2 L21 L26 L54 L55 L56 | L2 L20 L21 L26 L28 L29 L53 L54 L56 | L4 L5 L6 L7 L8 L9 | L10 L11 L12 L13 L14 L15 bodies 6 in component "Mount"
extrude "Extrude3'" add sketch "Sketch16" against normal blind 8 contours L2 L20 L23 L26 L27 L28 L49 L50 L52 | L2 L20 L26 L28 L50 L54 | L2 L20 L21 L26 L28 L29 L53 L54 L56 bodies 6 in component "Mount"
extrude "Extrude4'" add sketch "Sketch16" along normal blind 20 contours L0 L3 L23 L32 L46 L47 L48 | L0 L22 L23 L30 L31 L32 L45 L46 L48 | L0 L1 L21 L32 L42 L43 L44 | L0 L21 L22 L30 L32 L33 L41 L42 L44 | L2 L3 L23 L26 L50 L51 L52 | L2 L20 L23 L26 L27 L28 L49 L50 L52 | L1 L2 L21 L26 L54 L55 L56 | L2 L20 L21 L26 L28 L29 L53 L54 L56 bodies 6 in component "Mount"
ref_plane "WorkPlane1" through (-42, 17, 19.5) normal (-0.996195, -0.087156, 0) x (0, 0, -1)
split "Split3" by plane through (-42, 17, 19.5) normal (-0.996195, -0.087156, 0) bodies 6 makes body 7 at (-42, -13.6667, -18.6667) makes body 8 at (-42, 15.3333, 20.3333) makes body 9 at (-42, -15.3333, 20.3333) makes body 10 at (-42, 15.3333, -20.3333) in component "Mount"
delete_body "RemoveBody1" bodies 7 in component "Mount"
delete_body "RemoveBody2" bodies 8 in component "Mount"
delete_body "RemoveBody3" bodies 10 in component "Mount"
delete_body "RemoveBody4" bodies 9 in component "Mount"
ref_plane "WorkPlane2" through (-39.2441, -14.5, 22) normal (-0.98106, -0.085832, -0.173648) x (-0.087156, 0.996195, 0)
split "Split5" by plane through (-39.2441, -14.5, 22) normal (-0.98106, -0.085832, -0.173648) bodies 6 makes body 11 at (-39.317, -13.6667, 20.3333) makes body 12 at (-41.7084, 13.6667, 18.6667) makes body 13 at (-36.5164, 13.6667, -22) makes body 14 at (-36.721, -13.6667, -22) in component "Mount"
delete_body "RemoveBody5" bodies 11 in component "Mount"
delete_body "RemoveBody6" bodies 12 in component "Mount"
delete_body "RemoveBody7" bodies 13 in component "Mount"
delete_body "RemoveBody8" bodies 14 in component "Mount"
sketch "Sketch17" plane through (-35.2447, -3.0835, -6.2383) normal (-0.98106, -0.085832, -0.173648) x (0.087156, -0.996195, 0)
  line L0 (8.5149, 28.674) -> (8.5921, 23.5968)
  line L1 (8.5921, 23.5968) -> (13.6112, 23.5968)
  line L2 (13.6112, 23.5968) -> (13.534, 28.674)
  line L3 (13.534, 28.674) -> (8.5149, 28.674)
  line L4 (13.534, 28.674) -> (-20.5783, 28.674)
  line L5 (-20.5783, 28.674) -> (-19.9004, -15.9479)
  line L6 (-19.9004, -15.9479) -> (14.2058, -15.9479)
  line L7 (14.2058, -15.9479) -> (13.534, 28.674)
  constraint coincident L2.end L3.start
  constraint parallel L3 L4
  constraint parallel L2 L5
  constraint parallel L4 L6
extrude "Extrude5'" add sketch "Sketch17" along normal blind 2 bodies 6 in component "Mount"
sketch "Sketch19" plane through (-22, 0, 0) normal (1, 0, 0) x (0, 1, 0)
  line L0 (-17, -20) -> (17, -20)
  line L1 (17, -20) -> (17, 20)
  line L2 (17, 20) -> (-17, 20)
  line L3 (-17, 20) -> (-17, -20)
  line L4 (-7.664, 15.1819) -> (7.664, 15.1819)
  line L5 (7.664, 15.1819) -> (7.664, -2.9908)
  line L6 (7.664, -2.9908) -> (-7.664, -2.9908)
  line L7 (-7.664, -2.9908) -> (-7.664, 15.1819)
  line L8 (-7.664, -2.9908) -> (7.664, -2.9908)
  line L9 (7.664, -2.9908) -> (7.664, -16.7445)
  line L10 (7.664, -16.7445) -> (-7.664, -16.7445)
  line L11 (-7.664, -16.7445) -> (-7.664, -2.9908)
  constraint horizontal L8
  constraint vertical L9
  constraint horizontal L10
  constraint vertical L11
  constraint coincident L6.end L7.start
extrude "Extrude6'" cut sketch "Sketch19" against normal blind 3 contours L6 L8 L9 L10 L11 bodies 6 in component "Mount"
sketch "Sketch21" plane through (-37.2068, -3.2552, -6.5856) normal (-0.98106, -0.085832, -0.173648) x (0.087156, -0.996195, 0)
  line L0 (14.2058, -15.9479) -> (13.534, 28.674)
  line L1 (13.534, 28.674) -> (-20.5783, 28.674)
  line L2 (-20.5783, 28.674) -> (-19.9004, -15.9479)
  line L3 (-19.9004, -15.9479) -> (14.2058, -15.9479)
  line L4 (13.534, 28.674) -> (-19.9004, -15.9479)
  line L5 (14.2058, -15.9479) -> (-20.5783, 28.674)
  line L6 (-3.5221, 28.674) -> (-2.8473, -15.9479)
  circle A0 centre (-2.9879, -6.6493) radius 1.75
  circle A1 centre (-3.2801, 12.6704) radius 1.75
  dimension "d168" = 3.5
  dimension "d169" = 3.5
  constraint coincident L0.end L1.start
  constraint coincident L2.end L3.start
  constraint coincident L0.start L3.end
  constraint coincident L1.end L2.start
  constraint midpoint L1 L6.start
  constraint midpoint L3 L6.end
  constraint coincident L6 A0.centre
  constraint coincident L6 A1.centre
  measures "d168" diameter of A0
  measures "d169" diameter of A1
extrude "Extrude7" cut sketch "Sketch21" against normal blind 2 contours L6 A0 | L6 A0 | L6 A1 | L6 A1 bodies 6 in component "Mount"
split "Split4" by plane through (-39.2441, -14.5, 22) normal (-0.98106, -0.085832, -0.173648) bodies 6 makes body 15 at (-39.9614, 11.7053, 1.5819) in component "Mount"
sketch "Sketch22" plane through (0, 0, 22) normal (0, 0, 1) x (-1, 0, 0)
  line L0 (42, -17) -> (41.5626, -12)
  line L1 (41.5626, -12) -> (24, -12)
  line L2 (24, -12) -> (24, 12)
  line L3 (24, 12) -> (39.4628, 12)
  line L4 (39.4628, 12) -> (39.0254, 17)
  line L5 (39.0254, 17) -> (14, 17)
  line L6 (14, 17) -> (14, -17)
  line L7 (14, -17) -> (42, -17)
  line L8 (15.9966, 0) -> (20.001, 0)
  circle A0 centre (17.9988, 0) radius 1.75
  dimension "d172" = 3.5
  constraint perpendicular L2 L8
  constraint midpoint L8 A0.centre
  measures "d172" diameter of A0
extrude "Extrude8'" cut sketch "Sketch22" against normal blind 2 contours L8 A0 | L8 A0 bodies 6 in component "Mount"
sketch "Sketch23" plane through (0, 0, -22) normal (0, 0, -1) x (1, 0, 0)
  line L0 (-31.2374, 17) -> (-31.6748, 12)
  line L1 (-31.6748, 12) -> (-24, 12)
  line L2 (-24, 12) -> (-24, -12)
  line L3 (-24, -12) -> (-33.7745, -12)
  line L4 (-33.7745, -12) -> (-34.212, -17)
  line L5 (-34.212, -17) -> (-14, -17)
  line L6 (-14, -17) -> (-14, 17)
  line L7 (-14, 17) -> (-31.2374, 17)
  line L8 (-20.0104, -0.0104) -> (-15.9997, -0.0104)
  circle A0 centre (-18.005, -0.0104) radius 1.75
  dimension "d175" = 3.5
  constraint horizontal L8
  constraint midpoint L8 A0.centre
  measures "d175" diameter of A0
extrude "Extrude9'" cut sketch "Sketch23" against normal blind 2 contours L8 A0 | L8 A0 bodies 6 in component "Mount"
fillet "Fillet1'" radius 12.5 4 edges at (-14, 17, 21) (-14, 17, -21) (-14, -17, -21) (-14, -17, 21) on bodies 6 in component "Mount"
combine "Combine1" operation add target body 6 tool bodies 15 in component "Mount"
extrude "Extrude10'" cut 1 faces at (-21.2517, 0.0035, -20) along direction (0, 0, -1) blind 0.2 on bodies 6 bodies 6 in component "Mount"
extrude "Extrude11'" cut 1 faces at (-21.2496, 0, 20) along direction (0, 0, 1) blind 0.2 on bodies 6 bodies 6 in component "Mount"
component "Rear" placed x (1, 0, 0) y (0, 1, 0) z (0, 0, 1) at (0, 0, 0)
component "Front" placed x (1, 0, 0) y (0, 1, 0) z (0, 0, 1) at (0, 0, 0)
component "Mount" placed x (1, 0, 0) y (0, 1, 0) z (0, 0, 1) at (0, 0, 0)
named bodies: "Front", "Rear", "Mounting Frame", "Mounting Frame (4)", "Mounting Frame (1)", "Mounting Frame (2)", "Mounting Frame (3)"
